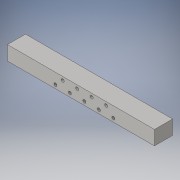
# Autodesk Inventor part: Block
Saved by Autodesk Inventor 2016 (Build 200138000, 138)
## iProperties
Created: 2015-04-25
Part Number: Block
Material: Aluminum 6061
Document SubType Name: Modeling
Designer: Atok
Density: 2.7 g/cm^3
Appearance: Aluminum - Flat
Mass: 4295.22 g
Surface Area: 1411.36 cm^2
Volume: 1590.82 cm^3
Author: Atok
Autodesk Inventor part; units mm, degrees
ref_plane "YZ Plane" through (0, 0, 0) normal (1, 0, 0) x (0, 1, 0)
ref_plane "XZ Plane" through (0, 0, 0) normal (0, 1, 0) x (-1, 0, 0)
ref_plane "XY Plane" through (0, 0, 0) normal (0, 0, 1) x (1, 0, 0)
derived "Blade.ipt"
sketch "Sketch10" plane through (0, 0, 3.048) normal (0, 0, 1) x (1, 0, 0)
  circle A0 centre (855.6691, 77) radius 5.3
  circle A1 centre (754.0691, 77) radius 5.3
  circle A2 centre (804.8691, 77) radius 5.3
  circle A3 centre (906.4691, 77) radius 5.3
  circle A4 centre (912.9603, 103.8139) radius 3.3
  circle A5 centre (889.5755, 125.2842) radius 3.3
  circle A6 centre (865.1509, 145.5652) radius 3.3
  circle A7 centre (839.8598, 164.7559) radius 3.3
  circle A8 centre (813.8348, 182.9396) radius 3.3
  circle A9 centre (787.1796, 200.1867) radius 3.3
  circle A10 centre (759.9766, 216.5567) radius 3.3
  circle A11 centre (732.293, 232.1005) radius 3.3
  circle A12 centre (704.1839, 246.8613) radius 3.3
  circle A13 centre (675.6958, 260.8767) radius 3.3
  circle A14 centre (646.8677, 274.1792) radius 3.3
  circle A15 centre (617.7334, 286.7971) radius 3.3
  circle A16 centre (588.3221, 298.7552) radius 3.3
  circle A17 centre (558.6594, 310.0756) radius 3.3
  circle A18 centre (528.768, 320.7776) radius 3.3
  circle A19 centre (498.6682, 330.8786) radius 3.3
  circle A20 centre (468.3782, 340.3941) radius 3.3
  circle A21 centre (437.9145, 349.3382) radius 3.3
  circle A22 centre (407.2922, 357.7232) radius 3.3
  circle A23 centre (376.5252, 365.5609) radius 3.3
  circle A24 centre (345.6263, 372.8614) radius 3.3
  circle A25 centre (314.6075, 379.6344) radius 3.3
  circle A26 centre (283.48, 385.8887) radius 3.3
  circle A27 centre (252.2541, 391.6322) radius 3.3
  circle A28 centre (220.9399, 396.8726) radius 3.3
  circle A29 centre (189.5467, 401.6167) radius 3.3
  circle A30 centre (158.0833, 405.8711) radius 3.3
  circle A31 centre (126.5584, 409.6419) radius 3.3
  circle A32 centre (94.9799, 412.9348) radius 3.3
  circle A33 centre (63.3557, 415.7554) radius 3.3
  circle A34 centre (31.6933, 418.1088) radius 3.3
  circle A35 centre (0, 420) radius 3.3
  line L0 (715.0844, 50) -> (711.797, 50)
  line L1 (1000, 0) -> (660.5382, 0)
  line L2 (974.7275, 50) -> (964.494, 50)
  line L3 (964.494, 50) -> (964.494, 65)
  line L4 (-40, 442.0963) -> (0, 440)
  line L5 (0, 400) -> (-40, 442.0963)
  line L6 (715.0844, 65) -> (715.0844, 50)
  circle A36 centre (906.4691, 38.1) radius 5.3
  circle A37 centre (804.8691, 38.1) radius 5.3
  circle A38 centre (881.0691, 12.7) radius 5.3
  circle A39 centre (779.4691, 12.7) radius 5.3
  circle A40 centre (830.2691, 12.7) radius 5.3
  circle A41 centre (728.6691, 12.7) radius 5.3
  circle A42 centre (931.8691, 12.7) radius 5.3
  circle A43 centre (855.6691, 38.1) radius 5.3
  circle A44 centre (754.0691, 38.1) radius 5.3
  spline S0 degree 3 poles (660.5382, 0) (843.9091, 84.4051) (554.1452, 370.9585) (0, 400) knots 1 1 1 1 2 2 2 2
  spline S1 degree 3 poles (0, 440) (549.2191, 411.2166) (932.7889, 184.6609) (1000, 0) knots 1 1 1 1 2 2 2 2
  spline S2 degree 3 poles (0, 440) (549.2191, 411.2166) (932.7889, 184.6609) (1000, 0) knots 1 1 1 1 2 2 2 2
  spline S3 degree 3 poles (660.5382, 0) (843.9091, 84.4051) (554.1452, 370.9585) (0, 400) knots 1 1 1 1 2 2 2 2
  point P0 (0, 0)
sketch "Sketch3" plane through (0, 0, 0) normal (0, 0, 1) x (1, 0, 0)
  circle A0 centre (906.4691, 38.1) radius 5.3 projected
  circle A1 centre (855.6691, 38.1) radius 5.3 projected
  circle A2 centre (804.8691, 38.1) radius 5.3 projected
  circle A3 centre (754.0691, 38.1) radius 5.3 projected
  circle A4 centre (728.6691, 12.7) radius 5.3 projected
  circle A5 centre (779.4691, 12.7) radius 5.3 projected
  circle A6 centre (830.2691, 12.7) radius 5.3 projected
  circle A7 centre (881.0691, 12.7) radius 5.3 projected
  circle A8 centre (931.8691, 12.7) radius 5.3 projected
  line L0 (559.397, 50) -> (1076.3275, 50)
  line L1 (1076.3275, 50) -> (1076.3275, 0)
  line L2 (1076.3275, 0) -> (559.397, 0)
  line L3 (559.397, 0) -> (559.397, 50)
  line L4 (0, 0) -> (1076.3275, 0) construction
  point P0 (711.797, 50)
  point P1 (974.7275, 50)
  dimension "d5" = 101.6
  dimension "d6" = 152.4
  constraints: 10 end point, 2 parallel, 2 perpendicular, 2 point on line, 1 collinear, 1 horizontal
  measures "d5" distance from line of point (974.727, 50) L1
  measures "d6" distance from line of point (711.797, 50) L3
extrude "Extrusion2" add sketch "Sketch3" along normal blind 63.5
body "Solid2"
